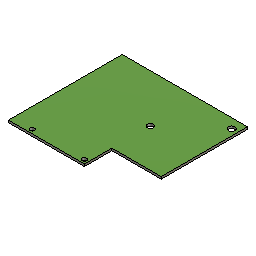
Teren Poarta Dreapta (Autodesk Fusion 360 design; units mm, degrees)
part number: 2026-06-02-22-18-47-467
Autodesk Fusion 360 part; units mm, degrees
note: some values were not read from the file. Set by a fixed rule: which sketch regions a step uses.
sketch "Sketch1" plane through (0, 0, 0) normal (0, 0, 1) x (1, 0, 0)
  line L0 (43.8447, -124.5942) -> (43.8447, 39.5803)
  line L1 (-67.5, 42.5803) -> (43.8447, 42.5803)
  line L2 (43.8447, 39.5803) -> (43.8447, 42.5803)
  circle A0 centre (38.3447, 34.0803) radius 5.5
  circle A1 centre (38.3447, 34.0803) radius 3
  line L3 (-67.5, 0) -> (-67.5, 39.5803)
  line L4 (-67.5, 39.5803) -> (-67.5, 42.5803)
  circle A2 centre (-50, 25) radius 3.5
  circle A3 centre (-50, 25) radius 2
  line L5 (-67.5, 0) -> (-67.5, -58.5)
  line L6 (0, -58.5) -> (-67.5, -58.5)
  circle A4 centre (-50, -55) radius 3.5
  circle A5 centre (-50, -55) radius 2
  circle A6 centre (-3.5, -55) radius 3.5
  circle A7 centre (-3.5, -55) radius 2
  line L7 (0, 0) -> (0, -55)
  line L8 (0, -55) -> (0, -58.5)
  line L9 (16.1782, -34.0942) -> (0, -34.0942)
  line L10 (16.1782, -34.0942) -> (34.5112, -34.0942)
  line L11 (34.5112, -34.0942) -> (43.8447, -34.0942)
  circle A8 centre (0, 0) radius 5.5
  circle A9 centre (0, 0) radius 2.75
extrude "Extrude1" add sketch "Sketch1" along normal blind 2 contours A0 | A4 | L0 L1 L2 L3 L4 L5 L6 A6 L7 L9 L10 L11 | A6 | L6 A6 L8 | A2 | A8
extrude "Extrude2" add sketch "Sketch1" along normal blind 1 contours A3
extrude "Extrude3" add sketch "Sketch1" against normal blind 5 contours A3
move_body "Move1" bodies 1 to x (1, 0, 0) y (0, 1, 0) z (0, 0, 1) at (0, 0, 130)
extrude "Extrude4" add 1 faces at (-51.1479, 25.5528, 131) along direction (0, 0, 1) blind 1
